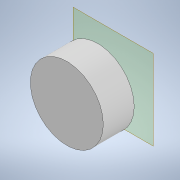
# Autodesk Inventor part: pots
Saved by Autodesk Inventor 2021 (Build 250183000, 183)
## iProperties
Created: 2021-07-12
Part Number: pots
Material: Generic
Document SubType Name: Modeling
Designer: Dell
Density: 1 g/cm^3
Appearance: Default
Author: Dell
Autodesk Inventor part; units mm, degrees
ref_plane "YZ Plane" through (0, 0, 0) normal (1, 0, 0) x (0, 1, 0)
ref_plane "XZ Plane" through (0, 0, 0) normal (0, 1, 0) x (-1, 0, 0)
ref_plane "XY Plane" through (0, 0, 0) normal (0, 0, 1) x (1, 0, 0)
sketch "Sketch1" plane through (0, 0, 0) normal (0, 0, 1) x (1, 0, 0)
  circle A0 centre (6.4435, 6.1377) radius 2.7646
  circle A1 centre (6.4435, 6.1377) radius 1.1803
  point P0 (0, 0)
  constraints: 2 centre point, 1 coincident
extrude "Extrusion1" add sketch "Sketch1" along normal blind 1 contours A1
ref_plane "Work Plane1" through (6.4435, 6.1377, -0.5) normal (0, 0, -1) x (-1, 0, 0)
sketch "Sketch2" plane through (6.4435, 6.1377, 0) normal (0, 0, -1) x (-1, 0, 0)
  circle A0 centre (0, 0) radius 0.5007
  point P0 (6.4435, -6.1377)
  constraints: 1 centre point
extrude "Extrusion2" add sketch "Sketch2" along normal blind 0.4
body "Solid1"
